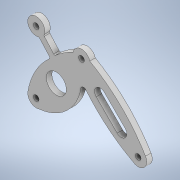
# Autodesk Inventor part: Final Bracket Design
Saved by Autodesk Inventor 2021 (Build 250183000, 183)
## iProperties
Created: 2021-05-08
Part Number: Final Bracket Design
Material: Generic
Document SubType Name: Modeling
Designer: Nabeel Azafer
Density: 1 g/cm^3
Appearance: Default
Author: Nabeel Azafer
Autodesk Inventor part; units mm, degrees
ref_plane "YZ Plane" through (0, 0, 0) normal (1, 0, 0) x (0, 1, 0)
ref_plane "XZ Plane" through (0, 0, 0) normal (0, 1, 0) x (-1, 0, 0)
ref_plane "XY Plane" through (0, 0, 0) normal (0, 0, 1) x (1, 0, 0)
sketch "Sketch1" plane through (0, 0, 0) normal (0, 0, 1) x (1, 0, 0)
  line L0 (-110.0561, 75) -> (109.9439, 75)
  line L1 (109.9439, 75) -> (109.9439, -75)
  line L2 (109.9439, -75) -> (-110.0561, -75)
  line L3 (-110.0561, -75) -> (-110.0561, 75)
  circle A0 centre (-90, 55) radius 5
  circle A1 centre (-90, -55) radius 5
  circle A2 centre (-10, 45.0091) radius 5
  circle A3 centre (90, -55) radius 5
  line L4 (-67, 0) -> (-42, 0)
  line L5 (-42, 0) -> (-42, -30) construction
  line L6 (-42, -30) -> (-67, -30) construction
  line L7 (-67, -30) -> (-67, 0) construction
  line L8 (40, -10) -> (59.9439, -10) construction
  line L9 (59.9439, -10) -> (59.9439, -30) construction
  line L10 (59.9439, -30) -> (40, -30) construction
  line L11 (40, -30) -> (40, -10) construction
  circle A4 centre (-54.5, -15) radius 10 construction
  ellipse E0 centre (-54.5, -15) end of major axis (-43.401, -1.5479) minor radius 17.7603
  circle A5 centre (43.0635, -13.1154) radius 3 construction
  circle A6 centre (47.4663, -17.5409) radius 3 construction
  circle A7 centre (51.9204, -22.0998) radius 3 construction
  circle A8 centre (56.7941, -26.2396) radius 3 construction
  circle A9 centre (-90, -55) radius 15
  arc A10 (-100.0358, -54.9482) -> (-100.0172, -55.6131) centre (-90, -55) ccw
  circle A11 centre (90.0005, -55.0001) radius 15
  line L12 (-85.4066, -69.2794) -> (85.4067, -69.2794) construction
  circle A12 centre (-10, 45.0091) radius 15
  line L13 (-24.261, 48.8375) -> (4.5032, 48.8375) construction
  arc A13 (102.8585, -47.2754) -> (4.5032, 48.8375) centre (-129.9643, -187.1488) ccw
  line L14 (-77.096, -62.6476) -> (77.0964, -62.6476) construction
  line L15 (81.0045, -67.0032) -> (-81.0042, -67.0032) construction
  line L16 (-14.3138, -6.5012) -> (6.7086, -6.5012) construction
  line L17 (-2.1245, 32.2429) -> (59.9439, -30) construction
  line L18 (59.9439, -30) -> (70.189, -40.245) construction
  arc A14 (-2.5267, 1.6589) -> (-10.9953, 0.4727) centre (-6.4015, -1.5012) ccw
  arc A15 (-2.5267, 1.6589) -> (81.0045, -67.0032) centre (209.7908, 174.8137) ccw
  line L19 (-65.2136, 18.8562) -> (-65.2134, 18.856)
  arc A16 (-24.6617, 48.1768) -> (-55.657, 27.7356) centre (42.7475, -87.7565) ccw
  arc A17 (-66.8653, 16.7082) -> (-104.7967, -52.539) centre (13.2065, -72.165) ccw
  line L20 (15.8581, 0.0478) -> (52.8629, -37.0611)
  line L21 (30.02, 14.1701) -> (67.0249, -22.9389)
  arc A18 (52.8828, -22.919) -> (52.8728, -22.9289) centre (59.9439, -30) ccw
  arc A19 (52.8629, -37.0611) -> (67.0249, -22.9389) centre (59.9439, -30) ccw
  arc A20 (-84.9219, -69.1143) -> (-10.9953, 0.4727) centre (-93.064, 13.5975) ccw
  arc A21 (30.02, 14.1701) -> (15.8581, 0.0478) centre (22.9391, 7.1089) ccw
  circle A22 centre (-90, 55) radius 15
  line L22 (-59.1413, 27.9714) -> (-75.7426, 46.5222)
  line L23 (-66.6758, 20.2327) -> (-84.0528, 39.6504)
  arc A23 (-66.8653, 16.7082) -> (-66.6758, 20.2327) centre (-68.5387, 18.5656) ccw
  arc A24 (-59.1413, 27.9714) -> (-55.657, 27.7356) centre (-57.2784, 29.6385) ccw
  arc A25 (-76.1826, 49.1623) -> (-75.7426, 46.5222) centre (-73.8797, 48.1894) ccw
  arc A26 (-84.0528, 39.6504) -> (-86.4992, 40.4142) centre (-85.9158, 37.9833) ccw
  point P0 (0, 0)
  point P1 (-6.3286, 6.5156)
  point P2 (-90, 71.308)
  point P3 (-104.5632, -51.4064)
  point P4 (-58.5353, 25.2193)
  point P5 (-108.4449, -75)
  point P6 (-76.3243, 48.8375)
  point P7 (34.0657, -6.0484)
  point P8 (-10.9953, 0.4727)
  dimension "d0" = 220
  dimension "d1" = 150
  dimension "d6" = 10
  dimension "d8" = 55
  dimension "d9" = 10
  dimension "d10" = 10
  dimension "d11" = 10
  dimension "d15" = 90
  dimension "d16" = 90
  dimension "d17" = 55
  dimension "d19" = 75
  dimension "d21" = 0
  dimension "d26" = 20
  dimension "d27" = 10
  dimension "d30" = 55
  dimension "d95" = 10
  dimension "d97" = 90
  dimension "d101" = 42
  dimension "d102" = 30
  dimension "d103" = 25
  dimension "d105" = 50
  dimension "d106" = 40
  dimension "d132" = 20
  dimension "d133" = 6
  dimension "d134" = 6
  dimension "d135" = 6
  dimension "d136" = 6
  dimension "d142" = 30
  dimension "d143" = 30
  dimension "d144" = 30
  dimension "d217" = 10
  dimension "d233" = 20
  dimension "d236" = 30
  dimension "d237" = 5
  dimension "d238" = 5
  dimension "d239" = 5
  dimension "d240" = 5
  constraints: 48 end point, 43 point on circle, 28 centre point, 14 tangent, 9 parallel, 6 coincident, 6 horizontal, 6 point on line, 3 perpendicular
  measures "d0" distance of L1.end L2.end
  measures "d1" distance of L2.end L0.start
  measures "d6" diameter of A0
  measures "d8" vertical distance of point (0, 0) A1.centre
  measures "d9" diameter of A1
  measures "d10" diameter of A3
  measures "d11" diameter of A2
  measures "d15" horizontal distance of point (0, 0) A3.centre
  measures "d16" horizontal distance of point (0, 0) A1.centre
  measures "d17" vertical distance of A0.centre point (0, 0)
  measures "d19" distance from line of point (0, 0) L0
  measures "d21" distance from line of point (0, 0) L4
  measures "d26" distance of L8.end L9.end
  measures "d27" distance from line of point (0, 0) L8
  measures "d30" vertical distance of point (0, 0) A3.centre
  measures "d95" horizontal distance of point (0, 0) A2.centre
  measures "d97" horizontal distance of point (0, 0) A0.centre
  measures "d101" distance from line of point (0, 0) L5
  measures "d102" distance of L6.end L4.start
  measures "d103" distance of L4.start L4.end
  measures "d105" distance between parallel lines of L1 L9
  measures "d106" distance from line of point (0, 0) L11
  measures "d132" diameter of A4
  measures "d133" diameter of A5
  measures "d134" diameter of A6
  measures "d135" diameter of A7
  measures "d136" diameter of A8
  measures "d142" diameter of A9
  measures "d143" diameter of A11
  measures "d144" diameter of A12
  measures "d217" diameter of A14
  measures "d233" diameter of A21
  measures "d236" diameter of A22
  measures "d237" diameter of A23
  measures "d238" diameter of A24
  measures "d239" diameter of A25
  measures "d240" diameter of A26
extrude "Extrusion39" add sketch "Sketch1" along normal blind 9.725 contours A9 | A9 A17 A23 L23 A26 A22 A25 L22 A24 A16 A12 A13 A11 A15 A14 A20 | A11 | A22 | A12
body "Solid38"
